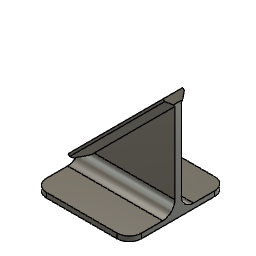
ROC_rev_C_screw_terminal_stand (Autodesk Fusion 360 design; units mm, degrees)
Autodesk Fusion 360 part; units mm, degrees
sketch "Sketch1" plane through (0, 0, 0) normal (0, 0, 1) x (1, 0, 0)
  line L0 (0, 0) -> (-3, 0)
  line L1 (-3, 0) -> (-38.8909, 0)
  line L2 (-38.8909, 0) -> (0, 38.8909)
  line L3 (0, 38.8909) -> (0, 0)
  dimension "d438" = 0
  dimension "d439" = 0
  dimension "d440" = 0
  dimension "d441" = 0
  dimension "d450" = 55
  dimension "d451" = 45
  dimension "d456" = 0
  dimension "d457" = 0
  dimension "d458" = 0
  dimension "d459" = 0
  constraint coincident L0.start L3.end
  constraint horizontal L0
  constraint parallel L0 L1
  constraint perpendicular L0 L3
  measures "d450" distance of L1.end L2.end
  measures "d451" angle of L1 L2
extrude "Extrude1" add sketch "Sketch1" along normal blind 2.6
ref_plane "WorkPlane1" through (-21.5668, 21.5668, 1.3) normal (-0.707107, 0.707107, 0) x (-0.707107, -0.707107, 0)
sketch "Sketch2" plane through (-21.5668, 21.5668, 1.3) normal (-0.707107, 0.707107, 0) x (-0.707107, -0.707107, 0)
  line L0 (-27.5, -4) -> (27.5, -4)
  line L1 (27.5, -4) -> (27.5, 4)
  line L2 (27.5, 4) -> (-27.5, 4)
  line L3 (-27.5, 4) -> (-27.5, -4)
  line L4 (-27.5, -4) -> (27.5, 4) construction
  line L5 (27.5, -4) -> (-27.5, 4) construction
  dimension "d453" = 55
  dimension "d464" = 8
  constraint horizontal L0
  constraint perpendicular L0 L1
  constraint parallel L0 L2
  constraint parallel L1 L3
  constraint coincident L4 origin
  constraint coincident L5 origin
  measures "d453" distance of L1 L3
  measures "d464" distance of L0 L2
extrude "Extrude2" add sketch "Sketch2" against normal up to surface (3 mm away)
chamfer "Chamfer1" distance 2.1 angle 45 2 edges at (-19.4454, 19.4454, -2.7) (-19.4454, 19.4454, 5.3)
sketch "Sketch4" plane through (19.4454, 19.4454, 0) normal (0.707107, 0.707107, 0) x (0, 0, -1)
  line L0 (-5.3, 29.6) -> (-3.2, 27.5)
  line L1 (-3.2, 27.5) -> (-2.6, 27.5)
  line L2 (-2.6, 27.5) -> (0, 27.5)
  line L3 (0, 27.5) -> (0.6, 27.5)
  line L4 (0.6, 27.5) -> (2.7, 29.6)
  line L5 (2.7, 29.6) -> (2.7, 30.5)
  line L6 (2.7, 30.5) -> (-5.3, 30.5)
  line L7 (-5.3, 30.5) -> (-5.3, 29.6)
  line L8 (0.6, 27.5) -> (0, 26.9)
  line L9 (0, 27.5) -> (0, 26.9)
  line L10 (-2.6, 27.5) -> (-2.6, 27.3)
  line L11 (-2.6, 27.3) -> (-2.6, 26.9)
  line L12 (-3.2, 27.5) -> (-2.6, 26.9)
  constraint coincident L3.end L4.start
  constraint parallel L4 L8
  constraint coincident L2.end L3.start
  constraint perpendicular L2 L9
  constraint coincident L1.end L2.start
  constraint perpendicular L2 L10
  constraint perpendicular L2 L11
  constraint coincident L0.end L1.start
  constraint parallel L0 L12
extrude "Extrude4" add sketch "Sketch4" along normal up to surface contours L1 L10 L11 L12 | L3 L8 L9 end surface through (0, 0, 0) normal (0, -1, 0) offset 0
sketch "Sketch5" plane through (0, 0, 2.6) normal (0, 0, 1) x (1, 0, 0)
  line L0 (0, 38.0423) -> (-38.0423, 0)
  line L1 (-38.0423, 0) -> (0, 0)
  line L2 (0, 0) -> (0, 38.0423)
  line L3 (0, 38.0423) -> (0, 38.8862)
  line L4 (0, 38.0423) -> (0.4219, 38.4643)
  line L5 (0.4219, 38.4643) -> (0, 38.8862)
  constraint coincident L0.start L2.end
  constraint parallel L2 L3
  constraint parallel L0 L4
  constraint perpendicular L4 L5
extrude "Extrude5" cut sketch "Sketch5" along normal mid plane 7 contours L3 L4 L5
extrude "Extrude6" cut 4 faces at (0.1414, 38.7479, 2.6) (0.1406, 38.7455, 2.7989) (0.1414, 38.7479, 0) (0.1406, 38.7455, -0.1989) along direction (0.707107, 0.707107, 0) blind 0.5
sketch "Sketch3" plane through (0, 0, 0) normal (0, -1, 0) x (1, 0, 0)
  line L0 (-38.0423, 0) -> (0, 0)
  line L1 (0, 0) -> (0, 2.6)
  line L2 (0, 2.6) -> (-38.0423, 2.6)
  line L3 (-38.8909, 3.2) -> (-38.8909, -0.6)
  line L4 (-38.8909, -18.6979) -> (0, -18.6979)
  line L5 (0, -18.6979) -> (0, 21.3021)
  line L6 (0, 21.3021) -> (-38.8909, 21.3021)
  line L7 (-38.8909, 21.3021) -> (-38.8909, -18.6979)
  line L8 (-38.8909, -18.6979) -> (0, 21.3021) construction
  line L9 (0, -18.6979) -> (-38.8909, 21.3021) construction
  line L10 (-38.0423, 2.6) -> (-38.8909, 3.2)
  line L11 (-38.8909, -0.6) -> (-38.0423, 0)
  line L12 (0, 2.6) -> (-38.8909, 0.0041)
  line L13 (0, 0) -> (-38.8909, 2.6014)
  point P0 (-19.4454, 1.3021)
  dimension "d466" = 40
  constraint horizontal L4
  constraint perpendicular L4 L5
  constraint parallel L4 L6
  constraint parallel L5 L7
  constraint coincident L8 P0
  constraint coincident L9 P0
  constraint collinear L3 L7
  constraint collinear L1 L5
  constraint coincident L1.end L2.start
  constraint coincident L7 L12.end
  constraint coincident L0.end L1.start
  constraint coincident L7 L13.end
  constraint midpoint P0 L12
  measures "d466" distance of L4.end L5.end
extrude "Extrude3" add sketch "Sketch3" along normal blind 2
fillet "Fillet2" radius 5 2 edges at (-19.0212, 0, 2.6) (-19.0212, 0, 0)
fillet "Fillet3" radius 5 4 edges at (-38.8909, -1, 21.3021) (0, -1, 21.3021) (0, -1, -18.6979) (-38.8909, -1, -18.6979)
